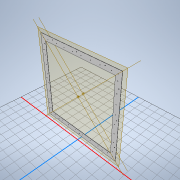
# Autodesk Inventor part: alu
Saved by Autodesk Inventor 2021 (Build 250183000, 183)
## iProperties
Created: 2021-06-22
Part Number: alu
Material: Aluminium 5052
Document SubType Name: Modeling
Designer: Wojciech Wołczek
Mass: 1619.36 g
Surface Area: 4242.74 cm^2
Volume: 604.238 cm^3
Density: 2.68 g/cm^3
Appearance: Satynowy — mocno szczotkowany
Author: Wojciech Wołczek
Autodesk Inventor part; units mm, degrees
ref_plane "YZ Plane" through (0, 0, 0) normal (1, 0, 0) x (0, 1, 0)
ref_plane "XZ Plane" through (0, 0, 0) normal (0, 1, 0) x (-1, 0, 0)
ref_plane "XY Plane" through (0, 0, 0) normal (0, 0, 1) x (1, 0, 0)
ref_plane "Płaszczyzna konstrukcyjna1" through (-413.1301, 496.4305, 6.8433) normal (0, 0, 1) x (0, -1, 0)
sketch "Szkic1" plane through (-413.1301, 496.4305, 6.8433) normal (0, 0, 1) x (0, -1, 0)
  line L0 (0, 905) -> (0, 0) projected
  line L1 (0, 0) -> (905, 0) projected
  line L2 (910, -5) -> (-5, -5) projected
  line L3 (-5, -5) -> (-5, 910) projected
  line L4 (-5, 910) -> (910, 910) projected
  line L5 (905, 905) -> (0, 905) projected
  line L6 (910, 910) -> (910, -5) projected
  line L7 (905, 0) -> (905, 905) projected
  line L8 (-6, -6) -> (911, -6)
  line L9 (911, -6) -> (911, 911)
  line L10 (911, 911) -> (-6, 911)
  line L11 (-6, 911) -> (-6, -6)
  line L12 (851, 54) -> (54, 54)
  line L13 (54, 54) -> (54, 851)
  line L14 (54, 851) -> (851, 851)
  line L15 (851, 851) -> (851, 54)
  point P0 (496.4305, 413.1301)
  dimension "d0" = 6
  dimension "d1" = 6
  dimension "d2" = 6
  dimension "d3" = 6
  dimension "d4" = 60
  constraints: 16 end point, 4 parallel, 2 perpendicular, 1 horizontal, 3 other
  measures "d0" distance between parallel lines of L0 L11
  measures "d1" distance between parallel lines of L1 L8
  measures "d2" distance between parallel lines of L7 L9
  measures "d3" distance between parallel lines of L5 L10
  measures "d4" distance between parallel lines of L8 L12
extrude "Wyciągnięcie proste1" add sketch "Szkic1" along normal blind 3 contours L5 L7 L1 L0 | L2 L3 L4 L6
sketch "Szkic2" plane through (-413.1301, 496.4305, 6.8433) normal (0, 0, -1) x (-1, 0, 0)
  line L0 (0, -905) -> (-905, -905) projected
  circle A0 centre (-452.5, -890) radius 4
  line L1 (-910, -910) -> (-910, 5) projected
  point P0 (-413.1301, -496.4305)
  dimension "d7" = 8
  dimension "d8" = 15
  dimension "d9" = 457.5
  constraints: 1 centre point
  measures "d7" diameter of A0
  measures "d8" distance from line of L0 A0.centre
  measures "d9" distance from line of L1 A0.centre
extrude "Wyciągnięcie proste2" cut sketch "Szkic2" against normal blind 10
pattern_linear "Szyk prostokątny1" count 2 spacing 300 along (1, 0, 0) count 2 spacing 300 along (-1, 0, 0) of "Wyciągnięcie proste2"
pattern_circular "Szyk kołowy1" count 4 over 360 about axis through (39.3699, 43.9305, 9.8433) along (0, 0, -1) of "Wyciągnięcie proste2", "Szyk prostokątny1"
sketch "Szkic3" plane through (-413.1301, 496.4305, 6.8433) normal (0, 0, -1) x (-1, 0, 0)
  line L0 (-770, -15) -> (-890, -15) projected
  line L1 (-890, -15) -> (-890, -135) projected
  arc A0 (-890, -170) -> (-890, -135) centre (-890, -152.5) ccw projected
  line L2 (-890, -170) -> (-890, -435) projected
  arc A1 (-890, -470) -> (-890, -435) centre (-890, -452.5) ccw projected
  line L3 (-890, -470) -> (-890, -735) projected
  arc A2 (-890, -770) -> (-890, -735) centre (-890, -752.5) ccw projected
  line L4 (-890, -770) -> (-890, -890) projected
  line L5 (-890, -890) -> (-770, -890) projected
  arc A3 (-735, -890) -> (-770, -890) centre (-752.5, -890) ccw projected
  line L6 (-735, -890) -> (-470, -890) projected
  arc A4 (-435, -890) -> (-470, -890) centre (-452.5, -890) ccw projected
  line L7 (-435, -890) -> (-170, -890) projected
  arc A5 (-135, -890) -> (-170, -890) centre (-152.5, -890) ccw projected
  line L8 (-135, -890) -> (-15, -890) projected
  line L9 (-15, -890) -> (-15, -770) projected
  arc A6 (-15, -735) -> (-15, -770) centre (-15, -752.5) ccw projected
  line L10 (-15, -735) -> (-15, -470) projected
  arc A7 (-15, -435) -> (-15, -470) centre (-15, -452.5) ccw projected
  line L11 (-15, -435) -> (-15, -170) projected
  arc A8 (-15, -135) -> (-15, -170) centre (-15, -152.5) ccw projected
  line L12 (-15, -135) -> (-15, -15) projected
  line L13 (-15, -15) -> (-135, -15) projected
  arc A9 (-170, -15) -> (-135, -15) centre (-152.5, -15) ccw projected
  line L14 (-170, -15) -> (-435, -15) projected
  arc A10 (-470, -15) -> (-435, -15) centre (-452.5, -15) ccw projected
  line L15 (-470, -15) -> (-735, -15) projected
  arc A11 (-770, -15) -> (-735, -15) centre (-752.5, -15) ccw projected
  circle A12 centre (-602.5, -30) radius 3 projected
  circle A13 centre (-815, -30) radius 3 projected
  circle A14 centre (-30, -30) radius 3 projected
  circle A15 centre (-502.5, -30) radius 3 projected
  circle A16 centre (-402.5, -30) radius 3 projected
  circle A17 centre (-30, -302.5) radius 3 projected
  circle A18 centre (-30, -90) radius 3 projected
  circle A19 centre (-30, -875) radius 3 projected
  circle A20 centre (-30, -402.5) radius 3 projected
  circle A21 centre (-30, -502.5) radius 3 projected
  circle A22 centre (-302.5, -875) radius 3 projected
  circle A23 centre (-90, -875) radius 3 projected
  circle A24 centre (-875, -875) radius 3 projected
  circle A25 centre (-402.5, -875) radius 3 projected
  circle A26 centre (-502.5, -875) radius 3 projected
  circle A27 centre (-875, -815) radius 3 projected
  circle A28 centre (-875, -30) radius 3 projected
  circle A29 centre (-875, -90) radius 3 projected
  circle A30 centre (-875, -202.5) radius 3 projected
  circle A31 centre (-875, -302.5) radius 3 projected
  circle A32 centre (-875, -402.5) radius 3 projected
  circle A33 centre (-875, -502.5) radius 3 projected
  circle A34 centre (-875, -602.5) radius 3 projected
  circle A35 centre (-875, -702.5) radius 3 projected
  circle A36 centre (-702.5, -875) radius 3 projected
  circle A37 centre (-602.5, -875) radius 3 projected
  circle A38 centre (-202.5, -875) radius 3 projected
  circle A39 centre (-815, -875) radius 3 projected
  circle A40 centre (-30, -702.5) radius 3 projected
  circle A41 centre (-30, -602.5) radius 3 projected
  circle A42 centre (-30, -202.5) radius 3 projected
  circle A43 centre (-30, -815) radius 3 projected
  circle A44 centre (-202.5, -30) radius 3 projected
  circle A45 centre (-302.5, -30) radius 3 projected
  circle A46 centre (-702.5, -30) radius 3 projected
  circle A47 centre (-90, -30) radius 3 projected
  point P0 (-413.1301, -496.4305)
extrude "Wyciągnięcie proste3" cut sketch "Szkic3" against normal blind 10 contours A12 | A13 | A14 | A15 | A16 | A17 | A18 | A19 | A20 | A21 | A22 | A23 | A24 | A25 | A26 | A27 | A28 | A29 | A30 | A31 | A32 | A33 | A34 | A35 | A36 | A37 | A38 | A39 | A40 | A41 | A42 | A43 | A44 | A45 | A46 | A47
